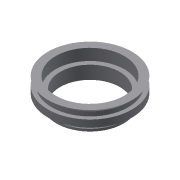
# Autodesk Inventor part: 101_Illumination_Adapter_Axiotech_COOLled
Saved by Autodesk Inventor 2019 (Build 230136000, 136)
## iProperties
Created: 2019-06-02
Part Number: 101_Illumination_Adapter_Axiotech_COOLled
Material: Generic
Document SubType Name: Modeling
Designer: diederichbenedict
Density: 1 g/cm^3
Appearance: Default
Author: diederichbenedict
Autodesk Inventor part; units mm, degrees
ref_plane "YZ Plane" through (0, 0, 0) normal (1, 0, 0) x (0, 1, 0)
ref_plane "XZ Plane" through (0, 0, 0) normal (0, 1, 0) x (-1, 0, 0)
ref_plane "XY Plane" through (0, 0, 0) normal (0, 0, 1) x (1, 0, 0)
sketch "Sketch1" plane through (0, 0, 0) normal (0, 0, 1) x (1, 0, 0)
  line L0 (0, 0) -> (0, 43.5277) construction
  line L1 (0, 0) -> (22, 0)
  line L2 (22, 0) -> (22, 1.5)
  line L3 (22, 1.5) -> (20.4, 3.1)
  line L4 (20.4, 3.1) -> (22, 4.7)
  line L5 (22, 4.7) -> (22, 6.1)
  line L6 (22, 6.1) -> (27.5, 6.1)
  line L7 (27.5, 6.1) -> (27.5, 10.7)
  line L8 (27.5, 10.7) -> (25, 10.7)
  line L9 (25, 10.7) -> (25, 13.5677)
  line L10 (25, 13.5677) -> (27.5, 16.0677)
  line L11 (25, 13.5677) -> (28.5355, 13.5677) construction
  line L12 (27.5, 16.0677) -> (22.5, 16.0677)
  line L13 (22.5, 16.0677) -> (22.5, 8.6)
  line L14 (22.5, 8.6) -> (19.5, 8.6)
  line L15 (19.5, 8.6) -> (19.5, 0)
  dimension "d0" = 22
  dimension "d1" = 1.5
  dimension "d2" = 135
  dimension "d3" = 90
  dimension "d4" = 3.2
  dimension "d5" = 1.4
  dimension "d6" = 6.1
  dimension "d7" = 27.5
  dimension "d8" = 4.6
  dimension "d10" = 45
  dimension "d11" = 5
  dimension "d12" = 2.5
  dimension "d13" = 2.5
  dimension "d14" = 2.5
  dimension "d15" = 2.5
  constraints: 32 end point, 5 horizontal, 5 perpendicular, 3 vertical, 2 point on line, 1 equal length
  measures "d0" distance of L0.start L1.end
  measures "d1" distance of L1.end L2.end
  measures "d2" angle of L3 L2
  measures "d3" angle of L3 L4
  measures "d4" distance of L2.end L4.end
  measures "d5" distance of L4.end L5.end
  measures "d6" distance of L1.end L5.end
  measures "d7" distance from line of L6.end L0
  measures "d8" distance of L6.end L7.end
  measures "d10" angle of L11 L10
  measures "d11" distance between parallel lines of L13 L7
  measures "d12" distance between parallel lines of L13 L9
  measures "d13" distance from line of L9.end L12
  measures "d14" distance between parallel lines of L14 L6
  measures "d15" distance between parallel lines of L15 L5
revolve "Revolution1" add sketch "Sketch1" angle 360 about axis through (0, 0, 0) along (0, 1, 0)
body "Solid1"
